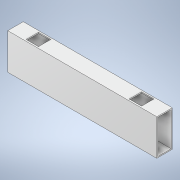
# Autodesk Inventor part: Travesaño
Saved by Autodesk Inventor 2022.6 (Build 266554000, 554)
## iProperties
Created: 2025-01-14
Part Number: Travesaño
Material: Genérico
Document SubType Name: Modeling
Designer: johan
Density: 1 g/cm^3
Appearance: Valor por defecto
Author: johan
Autodesk Inventor part; units mm, degrees
ref_plane "YZ Plane" through (0, 0, 0) normal (1, 0, 0) x (0, 1, 0)
ref_plane "XZ Plane" through (0, 0, 0) normal (0, 1, 0) x (-1, 0, 0)
ref_plane "XY Plane" through (0, 0, 0) normal (0, 0, 1) x (1, 0, 0)
sketch "Boceto1" plane through (0, 0, 0) normal (0, 1, 0) x (-1, 0, 0)
  line L0 (0, 0) -> (240, 0)
  line L1 (240, 0) -> (240, -25)
  line L2 (240, -25) -> (0, -25)
  line L3 (0, -25) -> (0, 0)
  dimension "d0" = 240
  dimension "d1" = 25
  constraints: 8 end point, 2 parallel, 1 horizontal, 1 perpendicular
  measures "d0" distance of L1.end L2.end
  measures "d1" distance of L0.end L1.end
extrude "Extrusión1" add sketch "Boceto1" along normal blind 58
sketch "Boceto2" plane through (0, 58, 0) normal (0, 1, 0) x (1, 0, 0)
  line L0 (0, 25) -> (-240, 25) projected
  line L1 (-240, 25) -> (-240, 0) projected
  line L2 (-240, 0) -> (0, 0) projected
  line L3 (0, 0) -> (0, 25) projected
  line L4 (-213, 2.5) -> (-193, 2.5)
  line L5 (-193, 2.5) -> (-193, 22.5)
  line L6 (-193, 22.5) -> (-213, 22.5)
  line L7 (-213, 22.5) -> (-213, 2.5)
  line L8 (-213, 2.5) -> (-193, 22.5) construction
  line L9 (-193, 2.5) -> (-213, 22.5) construction
  line L10 (-27, 22.5) -> (-47, 22.5)
  line L11 (-47, 22.5) -> (-47, 2.5)
  line L12 (-47, 2.5) -> (-27, 2.5)
  line L13 (-27, 2.5) -> (-27, 22.5)
  line L14 (-27, 22.5) -> (-47, 2.5) construction
  line L15 (-47, 22.5) -> (-27, 2.5) construction
  point P0 (-203, 12.5)
  point P1 (-37, 12.5)
  dimension "d10" = 20
  dimension "d11" = 20
  dimension "d12" = 20
  dimension "d13" = 20
  dimension "d14" = 27
  dimension "d15" = 146
  constraints: 24 end point, 4 midpoint, 4 parallel, 2 horizontal, 2 perpendicular
  measures "d10" distance of L6.end L5.end
  measures "d11" distance of L5.end L4.end
  measures "d12" distance of L12.end L11.end
  measures "d13" distance of L11.end L10.end
  measures "d14" distance between parallel lines of L13 L3
  measures "d15" distance between parallel lines of L5 L11
extrude "Extrusión2" cut sketch "Boceto2" against normal blind 58 contours L7 L6 L5 L4 | L13 L12 L11 L10
sketch "Boceto3" plane through (0, 0, 0) normal (1, 0, 0) x (0, 0, -1)
  line L0 (0, 0) -> (25, 0) projected
  line L1 (25, 0) -> (25, 58) projected
  line L2 (0, 58) -> (25, 58) projected
  line L3 (0, 0) -> (0, 58) projected
  line L4 (0, 0) -> (0, 58) projected
  line L5 (1.7, 52.5054) -> (1.7, 56.3)
  line L6 (1.7, 56.3) -> (23.3, 56.3)
  line L7 (25, 0) -> (25, 58) projected
  line L8 (22.5, 0) -> (2.5, 0) projected
  line L9 (7.4249, 0) -> (7.4249, 1.7)
  line L10 (7.4249, 1.7) -> (1.7, 1.7)
  line L11 (1.7, 52.5054) -> (1.7, 1.7)
  line L12 (7.4249, 1.7) -> (23.3, 1.7)
  line L13 (23.3, 1.7) -> (23.3, 56.3)
  point P0 (12.9, 29.7431)
  point P1 (2.5, 58)
  constraints: 14 end point, 3 perpendicular, 1 horizontal, 1 point on line, 1 vertical
extrude "Extrusión3" cut sketch "Boceto3" against normal blind 240 contours L5 L6 L13 L12 L10 L11
